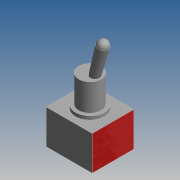
# Autodesk Inventor part: F112Interrupteur
Saved by Autodesk Inventor 2015 SP1 (Build 190203100, 203)
## iProperties
Created: 2017-01-26
Part Number: F112Interrupteur
Material: Générique
Document SubType Name: Modeling
Designer: serge.amoos
Density: 1 g/cm^3
Appearance: Par défaut
Author: serge.amoos
Autodesk Inventor part; units mm, degrees
ref_plane "YZ Plane" through (0, 0, 0) normal (1, 0, 0) x (0, 1, 0)
ref_plane "XZ Plane" through (0, 0, 0) normal (0, 1, 0) x (-1, 0, 0)
ref_plane "XY Plane" through (0, 0, 0) normal (0, 0, 1) x (1, 0, 0)
sketch "Sketch1" plane through (0, 0, 0) normal (0, 0, 1) x (1, 0, 0)
  line L0 (-8.89, 0) -> (8.89, 0) construction
  line L1 (0, -8.05) -> (0, 8.05) construction
  line L2 (-6.35, 5.75) -> (6.35, 5.75)
  line L3 (6.35, 5.75) -> (6.35, -5.75)
  line L4 (6.35, -5.75) -> (-6.35, -5.75)
  line L5 (-6.35, -5.75) -> (-6.35, 5.75)
  point P0 (0, 0)
  point P1 (0, 5.75)
  point P2 (6.35, 0)
  dimension "d0" = 12.7
  dimension "d1" = 11.5
  constraints: 8 end point, 2 midpoint, 2 parallel, 2 point on line, 1 horizontal, 1 perpendicular
  measures "d0" distance of L2.start L2.end
  measures "d1" distance of L2.end L3.end
extrude "Extrusion1" add sketch "Sketch1" along normal blind 9.5
sketch "Sketch2" plane through (0, 0, 9.5) normal (0, 0, 1) x (1, 0, 0)
  circle A0 centre (0, 0) radius 4
  dimension "d4" = 8
  constraints: 1 centre point, 1 coincident
  measures "d4" diameter of A0
extrude "Extrusion2" add sketch "Sketch2" along normal blind 1
sketch "Sketch3" plane through (0, 0, 10.5) normal (0, 0, 1) x (1, 0, 0)
  circle A0 centre (0, 0) radius 3.1
  dimension "d7" = 6.2
  constraints: 1 centre point, 1 coincident
  measures "d7" diameter of A0
extrude "Extrusion3" add sketch "Sketch3" along normal blind 7.5
sketch "Sketch4" plane through (0, 0, 0) normal (0, 1, 0) x (-1, 0, 0)
  line L0 (8.89, 0) -> (-8.89, 0) construction
  line L1 (0, -3.6) -> (0, 21.6) construction
  line L2 (0, 13) -> (-4.5899, 30.1296) construction
  line L3 (3.1, 18) -> (-3.1, 18) construction
  line L4 (-1.2212, 17.5575) -> (-2.4088, 17.2393)
  line L5 (-2.4088, 17.2393) -> (-5.3768, 27.271)
  line L6 (-5.3768, 27.271) -> (-3.9279, 27.6593)
  line L7 (-3.9279, 27.6593) -> (-1.2212, 17.5575)
  point P0 (0, 0)
  point P1 (-1.3397, 18)
  point P2 (-2.6338, 18)
  dimension "d10" = 15
  dimension "d11" = 5
  dimension "d13" = 10
  dimension "d14" = 3
  dimension "d16" = 2.5
  constraints: 10 end point, 7 point on line, 2 perpendicular, 1 collinear
  measures "d10" angle of L1 L2
  measures "d11" distance from line of L3 L2.start
  measures "d13" distance from line of point (-1.34, 18) L6
  measures "d14" diameter of L5.end L2
  measures "d16" diameter of point (-2.634, 18) L2
revolve "Revolution1" add sketch "Sketch4" angle 360 about axis through (0, 0, 13) along (0.258819, 0, 0.9659258)
fillet "Fillet1" radius 1.4 1 edges at (2.479, 0, 28.0475)
body "Solid1"
